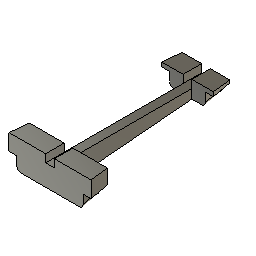
design (Autodesk Fusion 360 design; units mm, degrees)
Autodesk Fusion 360 part; units mm, degrees
note: some values were not read from the file. Set by a fixed rule: which face or edge a step refers to.
sketch "Sketch1" plane through (0, 0, 0) normal (0, 0, 1) x (1, 0, 0) in component "bottom"
  line L0 (0, 0) -> (0, -59) construction
  line L1 (-9.0108, 0) -> (9.0108, 0)
  line L2 (-15.5108, -59) -> (15.5108, -59)
  line L3 (-6, 0) -> (-12.5, -59)
  line L4 (6, 0) -> (12.5, -59)
  line L5 (-15.8315, -61.9115) -> (15.8315, -61.9115)
  line L6 (9.0108, 0) -> (15.8315, -61.9115)
  line L7 (-9.0108, 0) -> (9.0108, 0)
  line L8 (-9.0108, 0) -> (-15.8315, -61.9115)
  line L9 (1.65, 0) -> (1.65, -59)
  line L10 (-1.65, 0) -> (-1.65, -59)
  dimension "d1" = 12
  dimension "d2" = 25
  dimension "d3" = 59
  dimension "d64" = 3.3
  constraint vertical L0
  constraint horizontal L1
  constraint horizontal L2
  constraint equal L3 L4
  constraint coincident L6 L1.end
  constraint coincident L0.start L1
  constraint parallel L2 L5
  constraint parallel L4 L6
  constraint parallel L1 L7
  constraint parallel L3 L8
  constraint coincident L4.start L1
  constraint coincident L8 L1.start
  constraint coincident L3.start L1
  constraint coincident L6 L2.end
  constraint coincident L4.end L2
  constraint coincident L8 L2.start
  constraint coincident L3.end L2
  constraint symmetric L0 L3 L4
  constraint symmetric L0 L6 L8
  constraint coincident L0.start origin
  constraint coincident L7 L9.start
  constraint coincident L2 L9.end
  constraint perpendicular L2 L9
  constraint coincident L1 L10.start
  constraint coincident L2 L10.end
  constraint perpendicular L2 L10
  constraint symmetric L0 L9 L10
  measures "d1" distance of L3.start L4.start
  measures "d2" distance of L3.end L4.end
  measures "d3" distance of L1 L2
  measures "d64" distance of L9 L10
extrude "Extrude1" add sketch "Sketch1" along normal blind 1 contours L1 L2 L3 L7 L8 | L1 L2 L3 L7 L10 | L1 L2 L4 L7 L9 | L1 L2 L4 L6 L7 makes body 1 at (-8.7238, -39.3333, 0) makes body 2 at (8.7238, -39.3333, 0) in component "bottom"
extrude "Extrude2" add sketch "Sketch1" against normal blind 10 contours L1 L2 L3 L7 L10 | L1 L2 L7 L9 L10 | L1 L2 L4 L7 L9 bodies 1 2 in component "bottom"
extrude "Extrude3" cut sketch "Sketch1" against normal blind 2 contours L1 L2 L7 L9 L10 bodies 1 in component "bottom"
ref_plane "WorkPlane1" through (8.5804, -29.5, 1) normal (0, 0, 1) x (1, 0, 0) in component "bottom"
sketch "Sketch2" plane through (7.9054, -29.5, 1) normal (0, 0, 1) x (1, 0, 0) in component "bottom"
  line L0 (-23.4161, -29.5) -> (-9.5554, -29.5)
  line L1 (-9.5554, 29.5) -> (-16.9161, 29.5)
  line L2 (-16.9161, 29.5) -> (-23.4161, -29.5)
  line L3 (-6.2554, -29.5) -> (7.6054, -29.5)
  line L4 (7.6054, -29.5) -> (1.1054, 29.5)
  line L5 (1.1054, 29.5) -> (-6.2554, 29.5)
  line L6 (-16.9161, 29.5) -> (1.1054, 29.5)
  line L7 (-23.4161, -29.5) -> (7.6054, -29.5)
  line L8 (-17.6873, 22.5) -> (1.8766, 22.5)
  line L9 (-22.6449, -22.5) -> (6.8342, -22.5)
  line L10 (-9.5554, -29.5) -> (-9.5554, 29.5)
  line L11 (-6.2554, 29.5) -> (-6.2554, -29.5)
  dimension "d21" = 7
  dimension "d25" = 7
  constraint coincident L2 L8.start
  constraint coincident L4 L8.end
  constraint coincident L2 L9.start
  constraint coincident L4 L9.end
  constraint horizontal L9
  measures "d21" distance of L5 L8
  measures "d25" distance of L3 L9
extrude "Extrude7" cut sketch "Sketch2" against normal through all contours L2 L8 L9 L10 | L4 L8 L9 L11 bodies 1 in component "bottom"
sketch "Sketch1 (2)" plane through (0, 0, 0) normal (0, 0, 1) x (1, 0, 0) in component "top"
  line L0 (-4, 0) -> (4, 0)
  line L1 (-4, -30) -> (4, -30)
  line L2 (4, 0) -> (4, -30)
  line L3 (-4, 0) -> (-4, -30)
  line L4 (0, 0) -> (0, -100) construction
  line L5 (-12.5, 0) -> (12.5, 0)
  line L6 (12.5, 0) -> (12.5, -1)
  line L7 (12.5, -1) -> (-12.5, -1)
  line L8 (-12.5, -1) -> (-12.5, 0)
  line L9 (-4, -5) -> (4, -5)
  line L10 (-1.8, -5) -> (-1.8, -30)
  line L11 (1.8, -5) -> (1.8, -30)
  dimension "d36" = 8
  dimension "d37" = 30
  dimension "d39" = 1
  dimension "d40" = 25
  dimension "d41" = 5
  dimension "d42" = 3.6
  constraint horizontal L0
  constraint midpoint L4.start L0
  constraint horizontal L1
  constraint equal L0 L1
  constraint coincident L4.start origin
  constraint perpendicular L1 L4
  constraint coincident L1 L11.end
  constraint coincident L1 L10.end
  constraint horizontal L5
  constraint vertical L6
  constraint horizontal L7
  constraint vertical L8
  constraint midpoint L4.start L5
  constraint coincident L3 L9.start
  constraint coincident L2 L9.end
  constraint perpendicular L2 L9
  constraint coincident L9 L10.start
  constraint coincident L9 L11.start
  constraint symmetric L4 L10 L11
  measures "d36" distance of L0.start L0.end
  measures "d37" distance of L0 L1
  measures "d39" distance of L5 L7
  measures "d40" distance of L6 L8
  measures "d41" distance of L5 L9
  measures "d42" distance of L10 L11
extrude "Extrude1'" add sketch "Sketch1 (2)" along normal blind 8 separate body makes body 3 in component "top"
extrude "Extrude2'" cut sketch "Sketch1 (2)" along normal blind 6 contours L1 L9 L10 L11 bodies 3 in component "top"
ref_plane "WorkPlane1" through (0, -15, 8) normal (0, 0, 1) x (1, 0, 0) in component "top"
sketch "Sketch2 (2)" plane through (0, -15, 8) normal (0, 0, 1) x (1, 0, 0) in component "top"
  line L0 (-12.5, 15) -> (12.5, 15)
  line L1 (0, 15) -> (0, -85)
  line L2 (-2.25, 17.5) -> (2.25, 17.5)
  line L3 (2.25, 17.5) -> (2.25, 12.5)
  line L4 (2.25, 12.5) -> (-2.25, 12.5)
  line L5 (-2.25, 12.5) -> (-2.25, 17.5)
  line L6 (2.25, 17.5) -> (-2.25, 12.5) construction
  point P0 (0, 15)
  dimension "d48" = 4.5
  dimension "d49" = 5
  constraint horizontal L2
  constraint vertical L3
  constraint horizontal L4
  constraint vertical L5
  constraint midpoint P0 L6
  measures "d48" distance of L2.start L2.end
  measures "d49" distance of L2.start L4.end
extrude "Extrude3'" add sketch "Sketch2 (2)" along normal blind 5 bodies 3 in component "top"
chamfer "Chamfer1" distance 8 angle 45 2 edges at (-4, -1, 4) (4, -1, 4) on bodies 3 in component "top"
draft "Draft1" angle -30 neutral plane through (0, -2.5, 8) pull (0, -1, 0) 1 faces at (-0.75, 1.6667, 8) on bodies 3 in component "top"
fillet "Fillet1" radius 1 2 edges at (1.8, -17.5, 6) (-1.8, -17.5, 6) on bodies 3 in component "top"
fillet "Fillet2" radius 1.5 5 edges at (0, -30, 8) (-4, -19.5, 8) (4, -19.5, 8) (-4, -30, 4) (4, -30, 4) on bodies 3 in component "top"
fillet "Fillet3" radius 1 2 edges at (12.5, -1, 4) (-12.5, -1, 4) on bodies 3 in component "top"
chamfer "Chamfer2" distance 1.5 angle 45 2 edges at (2.25, -1.25, 8) (-2.25, -1.25, 8) on bodies 3 in component "top"
chamfer "Chamfer3" distance 1.5 angle 45 1 edges at (0, -2.5, 8) on bodies 3 in component "top"
draft "Draft3" angle -5 neutral plane through (-15.5108, -59, 0) pull (0, -1, 0) 1 faces at (-0.55, -56.6667, -10) on bodies 1 in component "bottom"
fillet "Fillet7" radius 1.5 4 edges at (6.3856, -3.5, -5.1444) (12.1144, -55.5, -9.6938) (-12.1144, -55.5, -9.6938) (-6.3856, -3.5, -5.1444) on bodies 1 in component "bottom"
draft "Draft4" angle 5 neutral plane through (-9.0108, 0, 0) pull (0, 1, 0) 4 faces at (7.2606, -2.3333, 0) (14.2501, -56.6667, 0) (-7.2606, -2.3333, 0) (-12.9895, -54.3333, 0) on bodies 1 in component "bottom"
fillet "Fillet9" [rolled back] radius 1 in component "bottom"
fillet "Fillet1'" [rolled back] radius 1 in component "bottom"
component "bottom" placed x (1, 0, 0) y (0, 1, 0) z (0, 0, 1) at (0, 0, 0)
component "top" placed x (1, 0, 0) y (0, 1, 0) z (0, 0, 1) at (0, 0, 0)
